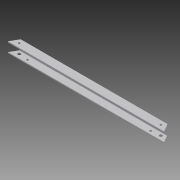
# Autodesk Inventor part: 19in c-channel-top
Saved by Autodesk Inventor 2013 (Build 170138000, 138)
## iProperties
Created: 2013-01-24
Part Number: 19in c-channel-top
Material: Generic
Document SubType Name: Modeling
Designer: Naphat
Density: 1 g/cm^3
Author: Naphat
Autodesk Inventor part; units mm, degrees
ref_plane "YZ Plane" through (0, 0, 0) normal (1, 0, 0) x (0, 1, 0)
ref_plane "XZ Plane" through (0, 0, 0) normal (0, 1, 0) x (-1, 0, 0)
ref_plane "XY Plane" through (0, 0, 0) normal (0, 0, 1) x (1, 0, 0)
sketch "Sketch1" plane through (0, 0, 0) normal (1, 0, 0) x (0, 1, 0)
  line L0 (-15.7, 12.7) -> (-12.7, 12.7)
  line L1 (-12.7, 12.7) -> (-12.7, -9.3)
  line L2 (-12.7, -9.3) -> (13.3, -9.3)
  line L3 (13.3, -9.3) -> (13.3, 13.1)
  line L4 (13.3, 13.1) -> (16.3, 13.1)
  line L5 (16.3, 13.1) -> (16.3, -12.3)
  line L6 (16.3, -12.3) -> (-15.7, -12.3)
  line L7 (-15.7, -12.3) -> (-15.7, 12.7)
  point P0 (0, 0)
  point P1 (0.3, 0.2)
  dimension "d0" = 3
  dimension "d1" = 3
  dimension "d2" = 25
  dimension "d3" = 32
  dimension "d4" = 16
  dimension "d5" = 12.5
  dimension "d6" = 3
  dimension "d44" = 22.4
  dimension "d45" = 16.3
  dimension "d46" = 13.1
  constraints: 16 end point, 6 parallel, 1 horizontal, 1 perpendicular
  measures "d0" distance of L0.start L0.end
  measures "d1" distance of L3.end L4.end
  measures "d2" distance of L6.end L0.start
  measures "d3" distance of L5.end L6.end
  measures "d4" distance from line of point (0.3, 0.2) L7
  measures "d5" distance from line of L6 point (0.3, 0.2)
  measures "d6" distance between parallel lines of L6 L2
  measures "d44" distance between parallel lines of L4 L2
  measures "d45" distance from line of point (0, 0) L5
  measures "d46" distance from line of point (0, 0) L4
extrude "Extrusion1" add sketch "Sketch1" along normal blind 482.6
sketch "Sketch3" plane through (0.7366, -15.7, 12.7) normal (0, -1, 0) x (1, 0, 0)
  line L0 (0, 0) -> (14.6558, -25.4) projected
  line L1 (-0.7366, -25) -> (481.8634, -25) projected
  line L2 (466.471, -25.4) -> (481.1268, 0) projected
  line L3 (-0.7366, 0) -> (481.8634, 0) projected
  line L4 (7.3279, -12.7) -> (473.7989, -12.7) construction
  line L5 (14.4316, 0) -> (28.8566, -25) construction
  circle A0 centre (21.6441, -12.5) radius 4.7625
  line L6 (466.6952, 0) -> (452.2702, -25) construction
  circle A1 centre (459.4827, -12.5) radius 4.7625
  point P0 (-0.7366, -12.7)
  dimension "d18" = 12.5
  dimension "d19" = 9.525
  dimension "d20" = 12.5
  dimension "d21" = 9.525
  constraints: 6 end point, 4 midpoint, 2 centre point, 2 parallel, 2 point on line, 3 other
  measures "d18" distance between parallel lines of L5 L0
  measures "d19" diameter of A0
  measures "d20" distance between parallel lines of L6 L2
  measures "d21" diameter of A1
hole "Access Hole" at (22.3807, -15.7, 0.2) at (460.2193, -15.7, 0.2) direction (0, 1, 0) diameter 9.525 depth 3 tip angle 118
sketch "Sketch4" plane through (0.7366, 16.3, 12.7) normal (0, 1, 0) x (1, 0, 0)
  circle A0 centre (21.6441, 12.5) radius 4.7625 projected
  circle A1 centre (459.4827, 12.5) radius 4.7625 projected
  circle A2 centre (21.6441, 12.5) radius 3.175
  circle A3 centre (459.4827, 12.5) radius 3.175
  point P0 (-0.7366, 12.7)
  dimension "d29" = 6.35
  dimension "d30" = 6.35
  constraints: 2 centre point, 2 coincident
  measures "d29" diameter of A2
  measures "d30" diameter of A3
hole "Mounting Hole" at (22.3807, 16.3, 0.2) at (460.2193, 16.3, 0.2) direction (0, -1, 0) diameter 6.35 depth 3 tip angle 118
chamfer "Chamfer1" distance 25 angle 30 1 edges at (0, 0.3, -12.3) measured on face at (0, 4.6333, -11.3)
chamfer "Chamfer2" distance 25 angle 30 1 edges at (482.6, 0.3, -12.3) measured on face at (482.6, 4.6333, -11.3)
sketch "Sketch5" plane through (0, -15.7, 12.7) normal (0, -1, 0) x (1, 0, 0)
  circle A0 centre (22.3807, -12.5) radius 4.7625 projected
  circle A1 centre (460.2193, -12.5) radius 4.7625 projected
  line L0 (0, 0) -> (482.6, 0) projected
  line L1 (14.4338, -25) -> (468.1662, -25) projected
  line L2 (51.0807, 0) -> (51.0807, -25) construction
  line L3 (431.5193, 0) -> (431.5193, -25) construction
  circle A2 centre (431.5193, -9.5) radius 3.175
  circle A3 centre (51.0807, -9.5) radius 3.175
  point P0 (0, -12.7)
  dimension "d47" = 28.7
  dimension "d49" = 28.7
  dimension "d61" = 6.35
  dimension "d62" = 15.5
  dimension "d63" = 6.35
  dimension "d71" = 51.0807
  constraints: 6 point on line, 4 end point, 2 centre point, 1 horizontal alignment, 1 parallel, 1 perpendicular
  measures "d47" distance from line of A0.centre L2
  measures "d49" distance from line of L3 A1.centre
  measures "d61" diameter of A2
  measures "d62" distance from line of L1 A2.centre
  measures "d63" diameter of A3
  measures "d71" distance from line of L0.start L2
hole "Hole4" at (51.0807, -15.7, 3.2) at (431.5193, -15.7, 3.2) direction (0, 1, 0) diameter 6.35 depth 3 tip angle 118
equation "\"d1\" = d0"
equation "\"d4\" = 0.5 * d3"
equation "\"d5\" = 0.5 * d2"
equation "\"d6\" = d0"
equation "\"d19\" = d21"
equation "\"d49\" = d47"
body "Solid1"
